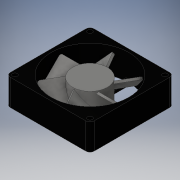
# Autodesk Inventor part: Lüfter
Saved by Autodesk Inventor 2016 (Build 200138000, 138)
## iProperties
Created: 2018-05-17
Part Number: Lüfter
Material: Generic
Document SubType Name: Modeling
Designer: Phil Erle
Density: 1 g/cm^3
Appearance: Default
Author: Phil Erle
Autodesk Inventor part; units mm, degrees
ref_plane "YZ Plane" through (0, 0, 0) normal (1, 0, 0) x (0, 1, 0)
ref_plane "XZ Plane" through (0, 0, 0) normal (0, 1, 0) x (-1, 0, 0)
ref_plane "XY Plane" through (0, 0, 0) normal (0, 0, 1) x (1, 0, 0)
sketch "Sketch1" plane through (0, 0, 0) normal (0, 0, 1) x (1, 0, 0)
  line L0 (-40, -40) -> (40, -40)
  line L1 (40, -40) -> (40, 40)
  line L2 (40, 40) -> (-40, 40)
  line L3 (-40, 40) -> (-40, -40)
  line L4 (-40, -40) -> (40, 40) construction
  line L5 (40, -40) -> (-40, 40) construction
  circle A0 centre (0, 0) radius 37
  dimension "d0" = 80
  dimension "d1" = 80
  dimension "d2" = 74
  constraints: 12 end point, 2 midpoint, 2 parallel, 1 centre point, 1 coincident, 1 horizontal, 1 perpendicular
  measures "d0" distance of L2.end L1.end
  measures "d1" distance of L1.end L0.end
  measures "d2" diameter of A0
extrude "Extrusion1" add sketch "Sketch1" along normal blind 25
sketch "Sketch2" plane through (0, 0, 25) normal (0, 0, 1) x (1, 0, 0)
  line L0 (-35.75, -35.75) -> (35.75, -35.75) construction
  line L1 (35.75, -35.75) -> (35.75, 35.75) construction
  line L2 (35.75, 35.75) -> (-35.75, 35.75) construction
  line L3 (-35.75, 35.75) -> (-35.75, -35.75) construction
  line L4 (-35.75, -35.75) -> (35.75, 35.75) construction
  line L5 (35.75, -35.75) -> (-35.75, 35.75) construction
  point P0 (0, 0)
  dimension "d5" = 71.5
  dimension "d6" = 71.5
  constraints: 12 end point, 4 coincident, 2 midpoint, 2 parallel, 1 horizontal, 1 perpendicular
  measures "d5" distance of L1.end L2.end
  measures "d6" distance of L0.end L1.end
hole "Hole1" at (-35.75, 35.75, 25) at (-35.75, -35.75, 25) at (35.75, -35.75, 25) at (35.75, 35.75, 25) direction (0, 0, -1) diameter 4.5 end through all clearance for "Countersunk Flat Head Screw DIN EN ISO 2009" size "M4" standard "DIN"
sketch "Sketch3" plane through (0, 0, 0) normal (0, 0, -1) x (-1, 0, 0)
  line L0 (40, -40) -> (-40, -40) projected
  line L1 (-2.5, -40) -> (2.5, -40)
  line L2 (2.5, -40) -> (2.5, -2.5)
  line L3 (2.5, -2.5) -> (40, -2.5)
  line L4 (40, 40) -> (40, -40) projected
  line L5 (40, -2.5) -> (40, 2.5)
  line L6 (40, 2.5) -> (2.5, 2.5)
  line L7 (2.5, 2.5) -> (2.5, 40)
  line L8 (2.5, 40) -> (-2.5, 40)
  line L9 (-2.5, 40) -> (-2.5, 2.5)
  line L10 (-2.5, 2.5) -> (-40, 2.5)
  line L11 (-40, 2.5) -> (-40, -2.5)
  line L12 (-40, -40) -> (-40, 40) projected
  line L13 (-40, -2.5) -> (-2.5, -2.5)
  line L14 (-2.5, -40) -> (-2.5, -2.5)
  point P0 (0, 0)
  point P1 (-40, 0)
  point P2 (40, 0)
  point P3 (0, -40)
  point P4 (0, 40)
  dimension "d14" = 5
  dimension "d15" = 5
  constraints: 24 end point, 12 point on line, 7 vertical alignment, 5 horizontal alignment, 5 perpendicular, 4 midpoint, 1 vertical
  measures "d14" distance between parallel lines of L2 L14
  measures "d15" distance between parallel lines of L13 L10
extrude "Extrusion2" add sketch "Sketch3" against normal blind 3 contours L0 L14 L13 L11 L10 L9 L8 L7 L6 L4 L3 L2
sketch "Sketch4" plane through (0, 0, 3) normal (0, 0, 1) x (1, 0, 0)
  circle A0 centre (0, 0) radius 16.5
  dimension "d18" = 33
  constraints: 1 centre point, 1 coincident
  measures "d18" diameter of A0
extrude "Extrusion3" add sketch "Sketch4" along normal blind 20
sketch "Sketch5" plane through (0, 0, 0) normal (1, 0, 0) x (0, 1, 0)
  line L0 (9.7071, 5.4142) -> (-6.8787, 22)
  line L1 (-6.8787, 22) -> (-8.2929, 20.5858)
  line L2 (-8.2929, 20.5858) -> (8.2929, 4)
  line L3 (8.2929, 4) -> (9.7071, 5.4142)
  line L4 (16.3095, 3) -> (36.9154, 3) projected
  line L5 (16.5, 23) -> (-16.5, 23) projected
  point P0 (0, 0)
  point P1 (0, 12.2929)
  dimension "d21" = 1
  dimension "d22" = 1
  dimension "d23" = 2
  dimension "d24" = 45
  constraints: 8 end point, 3 perpendicular, 1 midpoint, 1 vertical alignment
  measures "d21" distance from line of L2.end L4
  measures "d22" distance from line of L5 L0.end
  measures "d23" distance of L0.end L1.end
  measures "d24" angle of L4 L2
extrude "Extrusion4" add sketch "Sketch5" along normal blind 35
fillet "Fillet1" radius 2 2 edges at (35, -7.5858, 21.2929) (35, 9, 4.7071)
pattern_circular "Circular Pattern2" count 6 over 360 about axis through (0, 0, -10) along (0, 0, 1) of "Extrusion4", "Fillet1"
fillet "Fillet2" radius 4 4 edges at (40, -40, 12.5) (-40, -40, 12.5) (-40, 40, 12.5) (40, 40, 12.5)
body "Solid1"
